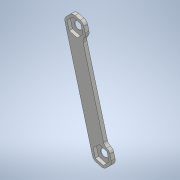
# Autodesk Inventor part: РельсКрышки
Saved by Autodesk Inventor 2020 (Build 240168000, 168)
## iProperties
Created: 2021-05-21
Part Number: РельсКрышки
Material: Типовые
Document SubType Name: Modeling
Designer: I_Love_U_Bogdan
Density: 1 g/cm^3
Appearance: По умолчанию
Author: I_Love_U_Bogdan
Autodesk Inventor part; units mm, degrees
ref_plane "YZ Plane" through (0, 0, 0) normal (1, 0, 0) x (0, 1, 0)
ref_plane "XZ Plane" through (0, 0, 0) normal (0, 1, 0) x (-1, 0, 0)
ref_plane "XY Plane" through (0, 0, 0) normal (0, 0, 1) x (1, 0, 0)
sketch "Эскиз1" plane through (0, 0, 0) normal (0, 0, 1) x (1, 0, 0)
  line L0 (-88.2272, -119.1) -> (-57.3625, -234.2883) projected
  line L1 (-71.2043, -171.0391) -> (-83.11, -126.6066) construction
  line L2 (-69.083, -167.3649) -> (-79.4357, -128.7279)
  line L3 (-85.2313, -130.2808) -> (-74.8785, -168.9178)
  arc A0 (-74.8785, -168.9178) -> (-69.083, -167.3649) centre (-71.9807, -168.1414) ccw
  arc A1 (-79.4357, -128.7279) -> (-85.2313, -130.2808) centre (-82.3335, -129.5043) ccw
  line L4 (-68.8409, -165.5636) -> (-67.9892, -168.7423)
  line L5 (-67.9892, -168.7423) -> (-70.3162, -171.0693)
  line L6 (-70.3162, -171.0693) -> (-73.495, -170.2176)
  line L7 (-73.495, -170.2176) -> (-74.3467, -167.0388)
  line L8 (-74.3467, -167.0388) -> (-72.0197, -164.7118)
  line L9 (-72.0197, -164.7118) -> (-68.8409, -165.5636)
  line L10 (-72.3186, -163.5965) -> (-75.4621, -166.74)
  line L11 (-75.4621, -166.74) -> (-74.3115, -171.0341)
  line L12 (-74.3115, -171.0341) -> (-70.0173, -172.1847)
  line L13 (-70.0173, -172.1847) -> (-66.8738, -169.0412)
  line L14 (-66.8738, -169.0412) -> (-68.0244, -164.7471)
  line L15 (-68.0244, -164.7471) -> (-72.3186, -163.5965)
  line L16 (-77.1571, -148.8229) -> (-74.2593, -148.0464)
  line L17 (-78.3254, -130.1669) -> (-79.1772, -126.9881)
  line L18 (-79.1772, -126.9881) -> (-82.356, -126.1364)
  line L19 (-82.356, -126.1364) -> (-84.683, -128.4634)
  line L20 (-84.683, -128.4634) -> (-83.8312, -131.6422)
  line L21 (-80.6525, -132.4939) -> (-78.3254, -130.1669)
  line L22 (-80.3536, -133.6093) -> (-84.6477, -132.4587)
  line L23 (-85.7983, -128.1645) -> (-82.6548, -125.021)
  line L24 (-82.6548, -125.021) -> (-78.3607, -126.1716)
  line L25 (-78.3607, -126.1716) -> (-77.2101, -130.4657)
  line L26 (-77.2101, -130.4657) -> (-80.3536, -133.6093)
  line L27 (-83.8312, -131.6422) -> (-80.6525, -132.4939)
  point P0 (0, 0)
  point P1 (-71.168, -167.8906)
  point P2 (-69.9205, -164.239)
  point P3 (-78.5981, -131.8538)
  dimension "d0" = 0
  dimension "d2" = 40
  dimension "d3" = 3
  dimension "d4" = 5.7
  dimension "d5" = 1
  dimension "d6" = 1
  constraints: 56 end point, 12 symmetric about line, 6 point on circle, 4 tangent, 2 centre point, 2 midpoint, 2 parallel, 2 point on line, 1 collinear, 18 other
  measures "d0" distance between parallel lines of L0 L3
  measures "d2" distance of A0.centre A1.centre
  measures "d3" radius of A0
  measures "d4" distance between parallel lines of L4 L7
  measures "d5" distance between parallel lines of L7 L3
  measures "d6" distance between parallel lines of L8 L10
extrude "Выдавливание1" add sketch "Эскиз1" along normal blind 2 contours L23 L24 L25 L26 L2 L21 L17 L18 L19 A1 L0 | A1 L19 L20 L27 L21 L2 L26 L22 L0 | L22 L26 L2 L15 L10 L0 | L10 L15 L2 L9 L8 L7 L6 A0 L0 | A0 L6 L5 L4 L9 L2 L15 L14 L13 L12 L0
sketch "Эскиз2" plane through (0, 0, 0) normal (0, 0, -1) x (-1, 0, 0)
  line L0 (78.3254, -130.1669) -> (80.6525, -132.4939) projected
  line L1 (84.683, -128.4634) -> (82.356, -126.1364) projected
  line L2 (83.8312, -131.6422) -> (84.683, -128.4634) projected
  line L3 (80.6525, -132.4939) -> (83.8312, -131.6422) projected
  line L4 (82.356, -126.1364) -> (79.1772, -126.9881) projected
  line L5 (79.1772, -126.9881) -> (78.3254, -130.1669) projected
  arc A0 (19.276, -252.9141) -> (17.0616, -251.2452) centre (19.4208, -250.4183) ccw projected
  arc A1 (19.276, -252.9141) -> (27.7531, -256.792) centre (35, -229.7461) ccw projected
  line L6 (48.5053, -262.3526) -> (27.7531, -256.792) projected
  line L7 (49.9977, -260.8602) -> (48.5053, -262.3526) projected
  arc A2 (51.783, -259.0748) -> (49.9977, -260.8602) centre (49.3645, -258.4417) ccw projected
  line L8 (60, -250.8579) -> (51.783, -259.0748) projected
  line L9 (60, -250.8579) -> (60, -245) projected
  line L10 (61.2941, -235.1704) -> (60, -245) projected
  line L11 (61.2941, -235.1704) -> (85, -146.6987) projected
  line L12 (85, -129.4867) -> (85, -146.6987) projected
  arc A3 (85, -111.5505) -> (85, -116.4495) centre (82.5, -114) ccw projected
  line L13 (85, -46.4495) -> (85, -111.5505) projected
  arc A4 (85, -41.5505) -> (85, -46.4495) centre (82.5, -44) ccw projected
  line L14 (85, -37.8284) -> (85, -41.5505) projected
  line L15 (76.4668, -29.2952) -> (85, -37.8284) projected
  arc A5 (72.9685, -21.4377) -> (76.4668, -29.2952) centre (84.9521, -20.8099) ccw projected
  arc A6 (72.9685, -21.4377) -> (27.398, -26.9013) centre (50, -22.641) ccw projected
  spline S0 degree 3 poles (27.6217, -27.9525) (27.5401, -27.6087) (27.4664, -27.263) (27.4007, -26.9157) (27.3998, -26.9109) (27.3989, -26.9061) (27.398, -26.9013) knots -4.945428 -4.945428 -4.945428 -4.945428 -4.899332 -4.899332 -4.899332 -4.898696 -4.898696 -4.898696 -4.898696 weights 1 1 1 1 1 1 1 projected
  spline S1 degree 3 poles (28.164, -30.4631) (27.9989, -29.614) (27.8171, -28.7759) (27.6217, -27.9525) knots 3.015096 3.015096 3.015096 3.015096 3.260421 3.260421 3.260421 3.260421 weights 1 1 1 1 projected
  spline S2 degree 3 poles (28.3854, -31.6677) (28.3156, -31.2645) (28.2417, -30.8629) (28.164, -30.4631) knots 1.901203 1.901203 1.901203 1.901203 2.021579 2.021579 2.021579 2.021579 projected
  spline S3 degree 3 poles (27.2821, -32.2702) (27.4905, -32.4048) (27.7033, -32.5146) (27.9524, -32.5655) (28.0203, -32.5713) (28.1301, -32.5543) (28.1726, -32.54) (28.2472, -32.4946) (28.2776, -32.4662) (28.335, -32.3905) (28.358, -32.3417) (28.403, -32.2042) (28.4139, -32.1072) (28.4174, -31.9004) (28.4051, -31.7812) (28.3854, -31.6677) knots 0 0 0 0 0.074448 0.074448 0.10037 0.10037 0.118258 0.118258 0.134856 0.134856 0.155747 0.155747 0.191916 0.191916 0.237121 0.237121 0.237121 0.237121 projected
  arc A7 (27.2821, -32.2702) -> (27.8696, -42.0032) centre (24, -37.3526) ccw projected
  spline S4 degree 3 poles (29.1017, -42.1691) (29.109, -42.0304) (29.1004, -41.9076) (29.061, -41.7446) (29.038, -41.6821) (28.9802, -41.5961) (28.9528, -41.5669) (28.8903, -41.5252) (28.8586, -41.5123) (28.7851, -41.4972) (28.7445, -41.4975) (28.6379, -41.5118) (28.5702, -41.5357) (28.3843, -41.6196) (28.2441, -41.7105) (28.0145, -41.8847) (27.9405, -41.9442) (27.8696, -42.0032) knots 0 0 0 0 0.041653 0.041653 0.066962 0.066962 0.083043 0.083043 0.096975 0.096975 0.113046 0.113046 0.139961 0.139961 0.194848 0.194848 0.220751 0.220751 0.220751 0.220751 projected
  spline S5 degree 3 poles (28.9908, -43.6688) (28.9918, -43.6586) (28.9927, -43.6484) (29.0398, -43.1514) (29.0756, -42.6615) (29.1017, -42.1691) knots 0.829158 0.829158 0.829158 0.829158 0.832223 0.832223 0.978679 0.978679 0.978679 0.978679 projected
  spline S6 degree 3 poles (19.7401, -60.1945) (21.5778, -59.1335) (23.1611, -57.7343) (25.061, -55.3244) (25.591, -54.5234) (27.536, -51.066) (28.3761, -48.1601) (28.7981, -45.2696) (28.876, -44.7357) (28.9396, -44.2038) (28.9908, -43.6688) knots 0 0 0 0 0.557778 0.557778 0.815105 0.815105 1.63021 1.63021 1.63021 1.780759 1.780759 1.780759 1.780759 weights 1 1 1 1 1 1 1 1 1 1 1 projected
  line L16 (19.7253, -60.203) -> (19.7401, -60.1945) projected
  line L17 (7, -67.55) -> (19.7253, -60.203) projected
  line L18 (7, -229.7461) -> (7, -67.55) projected
  arc A8 (7, -229.7461) -> (17.0616, -251.2452) centre (35, -229.7461) ccw projected
  circle A9 centre (27.4442, -220.4746) radius 2.5 projected
  circle A10 centre (38.4044, -239.4581) radius 7.5 projected
  circle A11 centre (24, -107.3526) radius 4 projected
  circle A12 centre (34.7265, -68.7944) radius 1.5 projected
  circle A13 centre (34.7265, -138.7944) radius 1.5 projected
  circle A14 centre (34.7265, -208.7944) radius 1.5 projected
  circle A15 centre (43.2836, -60.3339) radius 1.5 projected
  circle A16 centre (43.2836, -200.3339) radius 1.5 projected
  circle A17 centre (43.2836, -130.3339) radius 1.5 projected
  circle A18 centre (30.7187, -204.3292) radius 1.5 projected
  circle A19 centre (30.7187, -134.3292) radius 1.5 projected
  circle A20 centre (30.7187, -64.3292) radius 1.5 projected
  circle A21 centre (38.7342, -73.2595) radius 1.5 projected
  circle A22 centre (38.7342, -143.2595) radius 1.5 projected
  circle A23 centre (38.7342, -213.2595) radius 1.5 projected
  circle A24 centre (26.7109, -199.864) radius 1.5 projected
  circle A25 centre (26.7109, -129.864) radius 1.5 projected
  circle A26 centre (26.7109, -59.864) radius 1.5 projected
  circle A27 centre (50, -22.641) radius 6 projected
  circle A28 centre (24, -37.3526) radius 4 projected
  circle A29 centre (24, -177.3526) radius 4 projected
  circle A30 centre (57.3879, -228.498) radius 2.5 projected
  line L19 (74.3467, -167.0388) -> (72.0197, -164.7118) projected
  line L20 (73.495, -170.2176) -> (74.3467, -167.0388) projected
  line L21 (70.3162, -171.0693) -> (73.495, -170.2176) projected
  line L22 (67.9892, -168.7423) -> (70.3162, -171.0693) projected
  line L23 (68.8409, -165.5636) -> (67.9892, -168.7423) projected
  line L24 (72.0197, -164.7118) -> (68.8409, -165.5636) projected
  line L25 (80.6525, -132.4939) -> (83.8312, -131.6422) projected
  line L26 (79.1772, -126.9881) -> (78.3254, -130.1669) projected
  circle A31 centre (81.5042, -129.3151) radius 1.5
  circle A32 centre (71.168, -167.8906) radius 1.5
  arc A33 (85, -129.1436) -> (85, -129.4867) centre (81.5042, -129.3151) ccw projected
  line L27 (85, -116.4495) -> (85, -129.1436) projected
  circle A34 centre (71.168, -167.8906) radius 3.5 projected
  point P0 (0, 0)
  dimension "d9" = 3
  dimension "d10" = 3
  constraints: 2 centre point
  measures "d9" diameter of A31
  measures "d10" diameter of A32
extrude "Выдавливание2" add sketch "Эскиз2" against normal blind 0.2 contours L5 L4 L1 L2 L3 L0 | L20 L21 L22 L23 L24 L19
fillet "Сопряжение1" radius 2 10 edges at (-78.5981, -131.8538, 1) (-69.9205, -164.239, 1) (-68.0244, -164.7471, 1) (-66.8738, -169.0412, 1) (-70.0173, -172.1847, 1) (-74.3115, -171.0341, 1) (-82.6548, -125.021, 1) (-85.7983, -128.1645, 1) (-78.3607, -126.1716, 1) (-77.2101, -130.4657, 1)
